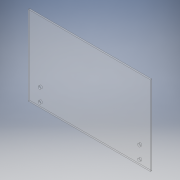
# Autodesk Inventor part: PaddleCollection2.1Backing
Saved by Autodesk Inventor 2019 (Build 230136000, 136)
## iProperties
Created: 2018-10-25
Part Number: PaddleCollection2.1Backing
Material: Polycarbonate, Clear
Document SubType Name: Modeling
Designer: User
Density: 1.2 g/cm^3
Appearance: Polycarbonate - Clear
Mass: 28.9054 g
Surface Area: 268.632 cm^2
Volume: 24.0878 cm^3
Author: User
Autodesk Inventor part; units mm, degrees
ref_plane "YZ Plane" through (0, 0, 0) normal (1, 0, 0) x (0, 1, 0)
ref_plane "XZ Plane" through (0, 0, 0) normal (0, 1, 0) x (-1, 0, 0)
ref_plane "XY Plane" through (0, 0, 0) normal (0, 0, 1) x (1, 0, 0)
sketch "Sketch1" plane through (0, 0, 0) normal (0, 0, 1) x (1, 0, 0)
  line L0 (0, 0) -> (152.4, 0)
  line L1 (152.4, 0) -> (152.4, 99.06)
  line L2 (152.4, 99.06) -> (0, 99.06)
  line L3 (0, 99.06) -> (0, 0)
  dimension "d0" = 152.4
  dimension "d1" = 99.06
  constraints: 8 end point, 2 parallel, 1 horizontal, 1 perpendicular
  measures "d0" distance of L2.end L1.end
  measures "d1" distance of L1.end L0.end
extrude "Extrusion1" add sketch "Sketch1" along normal blind 1.8542
sketch "Sketch2" plane through (0, 0, 1.8542) normal (0, 0, 1) x (1, 0, 0)
  line L0 (0, 99.06) -> (0, 0) projected
  line L1 (152.4, 99.06) -> (0, 99.06) projected
  line L2 (152.4, 0) -> (152.4, 99.06) projected
  point P0 (14.1478, 21.4884)
  point P1 (14.1478, 5.4884)
  point P2 (138.2522, 21.4884)
  point P3 (138.2522, 5.4884)
  dimension "d4" = 16
  dimension "d5" = 14.1478
  dimension "d6" = 14.1478
  dimension "d7" = 77.5716
  dimension "d8" = 16
  dimension "d9" = 14.1478
  dimension "d10" = 14.1478
  dimension "d11" = 77.5716
  measures "d4" distance of point (14.148, 5.488) point (14.148, 21.488)
  measures "d5" distance from line of point (14.148, 21.488) L0
  measures "d6" distance from line of L0 point (14.148, 5.488)
  measures "d7" distance from line of L1 point (14.148, 21.488)
  measures "d8" distance of point (138.252, 5.488) point (138.252, 21.488)
  measures "d9" distance from line of L2 point (138.252, 21.488)
  measures "d10" distance from line of L2 point (138.252, 5.488)
  measures "d11" distance from line of L1 point (138.252, 21.488)
hole "Hole1" at (14.1478, 21.4884, 1.8542) at (14.1478, 5.4884, 1.8542) at (138.2522, 21.4884, 1.8542) at (138.2522, 5.4884, 1.8542) direction (0, 0, -1) diameter 3.81 depth 10.9728 tip angle 118
equation "\"d6\" = d5"
equation "\"d8\" = d4"
equation "\"d9\" = d5"
equation "\"d10\" = d5"
equation "\"d11\" = d7"
body "Solid1"
